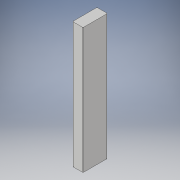
# Autodesk Inventor part: Wood 2x4x16
Saved by Autodesk Inventor 2019 (Build 230136000, 136)
## iProperties
Created: 2019-03-26
Part Number: Wood 2x4x16
Material: Generic
Document SubType Name: Modeling
Designer: torba
Density: 1 g/cm^3
Appearance: Default
Author: torba
Autodesk Inventor part; units mm, degrees
ref_plane "YZ Plane" through (0, 0, 0) normal (1, 0, 0) x (0, 1, 0)
ref_plane "XZ Plane" through (0, 0, 0) normal (0, 1, 0) x (-1, 0, 0)
ref_plane "XY Plane" through (0, 0, 0) normal (0, 0, 1) x (1, 0, 0)
sketch "Sketch1" plane through (0, 0, 0) normal (0, 1, 0) x (-1, 0, 0)
  line L0 (0, 0) -> (38.1, 0)
  line L1 (38.1, 0) -> (38.1, -88.9)
  line L2 (38.1, -88.9) -> (0, -88.9)
  line L3 (0, -88.9) -> (0, 0)
  dimension "d0" = 38.1
  dimension "d1" = 88.9
  constraints: 8 end point, 2 parallel, 1 horizontal, 1 perpendicular
  measures "d0" distance of L1.end L2.end
  measures "d1" distance of L0.end L1.end
extrude "Extrusion1" add sketch "Sketch1" along normal blind 457.2
sketch "Sketch2" plane through (0, 0, 0) normal (0, -1, 0) x (1, 0, 0)
  line L0 (0, -88.9) -> (-38.1, -88.9) projected
  line L1 (0, -88.9) -> (124.8054, 254)
  line L2 (0, -88.9) -> (364.9066, -88.9) construction
  line L3 (124.8054, 254) -> (47.8157, 298.45) construction
  line L4 (124.8054, 254) -> (213.7054, 254) construction
  line L5 (45.1457, 254) -> (-19.05, 77.6237)
  line L6 (47.8157, 298.45) -> (610.7445, 298.45) construction
  line L7 (-38.1, 0) -> (0, 0) projected
  line L8 (-19.05, 0) -> (-19.05, 77.6237)
  line L9 (124.8054, 254) -> (45.1457, 254)
  line L10 (124.8054, 254) -> (204.465, 254) construction
  dimension "d5" = 70
  dimension "d6" = 88.9
  dimension "d7" = 150
  dimension "d9" = 180
  dimension "d10" = 254
  dimension "d11" = 44.45
  dimension "d12" = 281.4644
  constraints: 18 end point, 4 horizontal, 3 equal length, 1 midpoint, 1 parallel, 1 vertical
  measures "d5" angle of L2 L1
  measures "d6" distance of L1.end L3.end
  measures "d7" angle of L4 L3
  measures "d9" angle of L9 L10
  measures "d10" distance between parallel lines of L7 L10
  measures "d11" distance from line of L7.end L5
  measures "d12" distance from line of L6.end L3
fillet "Fillet2" radius 3.175 4 edges at (0, 228.6, -88.9) (0, 228.6, 0) (-38.1, 228.6, -88.9) (-38.1, 228.6, 0)
body "Solid1"
